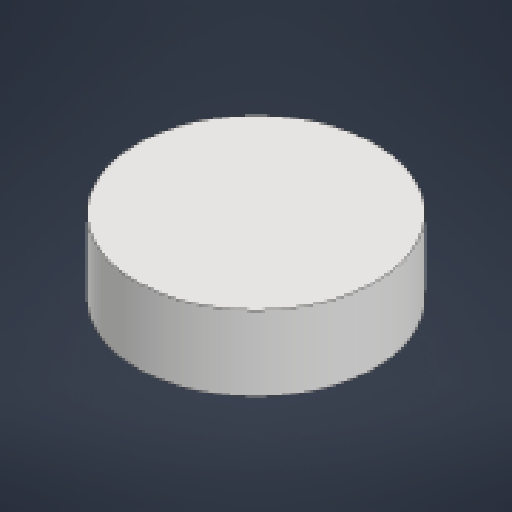
# Autodesk Inventor part: Standoff
Saved by Autodesk Inventor 2023 (Build 270158000, 158)
## iProperties
Created: 2023-02-16
Part Number: Standoff
Material: Generic
Document SubType Name: Modeling
Designer: Michael
Density: 1 g/cm^3
Appearance: Default
Author: Michael
Autodesk Inventor part; units mm, degrees
ref_plane "YZ Plane" through (0, 0, 0) normal (1, 0, 0) x (0, 1, 0)
ref_plane "XZ Plane" through (0, 0, 0) normal (0, 1, 0) x (-1, 0, 0)
ref_plane "XY Plane" through (0, 0, 0) normal (0, 0, 1) x (1, 0, 0)
ref_plane "Work Plane1" through (49.1494, -37.6525, 49.2967) normal (0, 1, 0) x (-1, 0, 0)
sketch "Sketch2" plane through (49.1494, -37.6525, 49.2967) normal (0, 1, 0) x (-1, 0, 0)
  line L0 (92.3663, -57.2126) -> (76.2, -41.0481) projected
  line L1 (92.3663, -57.2126) -> (69.9168, -79.6645) projected
  line L2 (53.7506, -63.5) -> (69.8965, -79.6442) projected
  line L3 (53.7506, -63.5) -> (76.2, -41.0481) projected
  line L4 (76.2, -41.0481) -> (92.3663, -57.2126)
  line L5 (92.3663, -57.2126) -> (69.8965, -79.6442)
  line L6 (69.8965, -79.6442) -> (53.7506, -63.5)
  line L7 (53.7506, -63.5) -> (76.2, -41.0481)
  point P0 (49.1494, -49.2967)
  constraints: 8 end point, 3 collinear
extrude "Extrusion2" add sketch "Sketch2" along normal blind 44.45
sketch "Sketch3" plane through (49.1494, 6.7975, 49.2967) normal (0, 1, 0) x (1, 0, 0)
  circle A0 centre (-77.0987, 52.7224) radius 2.4765 projected
  circle A1 centre (-65.425, 64.3974) radius 2.4765 projected
  point P0 (-49.1494, 49.2967)
  constraints: 2 coincident
hole "Hole1" at (-16.2756, 6.7975, -15.1007) at (-27.9493, 6.7975, -3.4258) direction (0, -1, 0) diameter 7.112 depth 10.414
sketch "Sketch4" plane through (49.1494, -37.6525, 49.2967) normal (0, -1, 0) x (1, 0, 0)
  circle A0 centre (-77.0987, -52.7224) radius 3.556 projected
  circle A1 centre (-65.425, -64.3974) radius 3.556 projected
  point P0 (-49.1494, -49.2967)
extrude "Extrusion3" cut sketch "Sketch4" against normal blind 10.414
fillet "Fillet1" radius 3.175 2 edges at (-20.7472, -15.4275, -30.3475) (-43.2169, -15.4275, -7.916)
body "Solid2"
